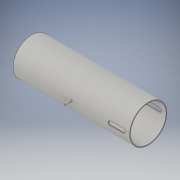
# Autodesk Inventor part: pitchingMachineTube
Saved by Autodesk Inventor 2016 SP1 (Build 200210100, 210)
## iProperties
Created: 2016-01-12
Part Number: pitchingMachineTube
Material: Generic
Document SubType Name: Modeling
Designer: steele
Density: 1 g/cm^3
Appearance: Default
Author: steele
Autodesk Inventor part; units mm, degrees
ref_plane "XZ Plane" through (0, 0, 0) normal (0, 1, 0) x (-1, 0, 0)
sketch "Sketch1" plane through (0, 0, 0) normal (1, 0, 0) x (0, 1, 0)
  circle A0 centre (0, 0) radius 139.7
  circle A1 centre (0, 0) radius 146.05
  dimension "d0" = 279.4
  dimension "d1" = 292.1
  constraints: 2 centre point, 2 coincident
  measures "d0" diameter of A0
  measures "d1" diameter of A1
extrude "Extrusion1" add sketch "Sketch1" along normal mid plane 914.4
ref_plane "Work Plane1" through (0, 0, 146.05) normal (0, 0, 1) x (1, 0, 0)
sketch "Sketch2" plane through (0, 0, 146.05) normal (0, 0, 1) x (1, 0, 0)
  circle A0 centre (0, 0) radius 6.35
  dimension "d4" = 12.7
  constraints: 1 centre point, 1 coincident
  measures "d4" diameter of A0
extrude "Extrusion2" add sketch "Sketch2" along normal blind 50.8
sketch "Sketch3" plane through (0, 0, 146.05) normal (0, 0, 1) x (1, 0, 0)
  line L0 (304.8, 0) -> (406.4, 0) construction
  line L1 (304.8, -15.875) -> (406.4, -15.875)
  line L2 (406.4, 15.875) -> (304.8, 15.875)
  arc A0 (304.8, 15.875) -> (304.8, -15.875) centre (304.8, 0) ccw
  arc A1 (406.4, -15.875) -> (406.4, 15.875) centre (406.4, 0) ccw
  line L3 (457.2, -146.05) -> (457.2, 146.05) projected
  point P0 (0, 0)
  point P1 (355.6, 0)
  dimension "d7" = 31.75
  dimension "d8" = 101.6
  dimension "d9" = 50.8
  constraints: 8 end point, 4 point on circle, 4 tangent, 2 centre point, 1 horizontal, 1 midpoint, 1 parallel
  measures "d7" distance between parallel lines of L1 L2
  measures "d8" distance of L0.end L0.start
  measures "d9" distance from line of L0.end L3
extrude "Extrusion3" cut sketch "Sketch3" against normal up to next
mirror "Mirror1" about plane through (0, 0, 0) normal (0, 0, 1) of "Extrusion3"
mirror "Mirror2" about plane through (0, 0, 0) normal (0, 0, 1) of "Extrusion2"
ref_plane "Work Plane3" through (355.6, 0, 0) normal (1, 0, 0) x (0, 1, 0)
equation "\"d0\" = pitchingMachineTubeDiam"
equation "\"d1\" = pitchingMachineOuterTubeDiam"
equation "\"d2\" = pitchingMachineTubeLength"
equation "\"d4\" = pitchingMachineTubeAxelDiam"
equation "\"d5\" = pitchingMachineTubeAxelLength"
equation "\"d7\" = pMTubeSlotWidth"
equation "\"d8\" = pMTubeSlotLength"
equation "\"d9\" = pMTubeSlotDistanceFromBack"
equation "\"d10\" = pitchingMachineTubeAxelLength"
equation "\"pitchingMachineTubeDiam\" = boulderDiam + boulderDiamVariation"
equation "\"boulderDiam\" = 254"
equation "\"boulderDiamVariation\" = 25.4"
equation "\"pitchingMachineTubeThickness\" = 6.35"
equation "\"pitchingMachineOuterTubeDiam\" = pitchingMachineTubeDiam + 2 * pitchingMachineTubeThickness"
equation "\"pitchingMachineTubeLength\" = 914.4"
equation "\"pitchingMachineTubeAxelDiam\" = 12.7"
equation "\"pitchingMachineTubeAxelLength\" = 50.8"
equation "\"pMTubeSlotLength\" = 101.6"
equation "\"pMTubeSlotWidth\" = 31.75"
equation "\"pMTubeSlotDistanceFromBack\" = 50.8"
equation "\"d13\" = pMTubeWheelDistanceFromBack"
equation "\"pMTubeWheelDistanceFromBack\" = 355.6"
body "Solid1"
